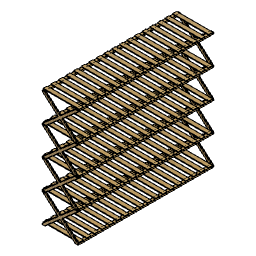
rgiro_akozlin_shelf (Autodesk Fusion 360 design; units mm, degrees)
Autodesk Fusion 360 part; units mm, degrees
note: some values were not read from the file. Chosen so that the rebuilt part matches the saved one: which bodies a step acts on. Set by a fixed rule: which face or edge a step refers to.
sketch "Sketch1" plane through (0, 0, 0) normal (0, 0, 1) x (1, 0, 0)
  line L0 (115, -500) -> (135, -500)
  line L1 (135, -500) -> (135, 500)
  line L2 (135, 500) -> (115, 500)
  line L3 (115, 500) -> (115, -500)
  line L4 (-135, -500) -> (-115, -500)
  line L5 (-115, -500) -> (-115, 500)
  line L6 (-115, 500) -> (-135, 500)
  line L7 (-135, 500) -> (-135, -500)
  dimension "d1" = 270
  dimension "d2" = 1000
  dimension "d4" = 20
  dimension "d7" = 135
  dimension "d29" = 500
  constraint horizontal L0
  constraint vertical L1
  constraint horizontal L2
  constraint vertical L3
  constraint horizontal L4
  constraint vertical L5
  constraint horizontal L6
  constraint vertical L7
  constraint equal L1 L7
  constraint equal L2 L6
  constraint collinear L2 L6
  measures "d1" distance of L1 L7
  measures "d2" distance of L4.start L6.end
  measures "d4" distance of L5.end L6.end
  measures "d7" distance of origin L1
  measures "d29" distance of origin L6
extrude "Extrude1" add sketch "Sketch1" along normal blind 10 makes body 1 at (121.6667, 166.6667, 0) makes body 2 at (-121.6667, 166.6667, 0)
sketch "Sketch2" plane through (0, 0, 10) normal (0, 0, 1) x (-1, 0, 0)
  line L0 (-115, -500) -> (-115, 500)
  line L1 (-115, 500) -> (-135, 500)
  line L2 (-135, 500) -> (-135, -500)
  line L3 (-135, -500) -> (-115, -500)
  line L4 (-135, 500) -> (135, 500)
  line L5 (135, 500) -> (135, 470)
  line L6 (135, 470) -> (-135, 470)
  line L7 (-135, 470) -> (-135, 500)
  line L8 (135, -500) -> (135, 500)
  dimension "d14" = 30
  constraint horizontal L4
  constraint vertical L5
  constraint horizontal L6
  constraint vertical L7
  constraint coincident L1.end L2.start
  constraint collinear L5 L8
  measures "d14" distance of L4.end L5.end
extrude "Extrude2" add sketch "Sketch2" along normal blind 5 separate body contours L0 L1 L2 L4 L6 L7 | L0 L4 L5 L6 L8 makes body 3
pattern_linear "R-Pattern3" count 18 spacing 57.0588 along (0, 1, 0) of bodies 3 makes body 4 at (31.6667, -432.9412, 10) makes body 5 at (31.6667, -375.8824, 10) makes body 6 at (31.6667, -318.8235, 10) makes body 7 at (31.6667, -261.7647, 10) makes body 8 at (31.6667, -204.7059, 10) makes body 9 at (31.6667, -147.6471, 10) makes body 10 at (31.6667, -90.5882, 10) makes body 11 at (31.6667, -33.5294, 10) makes body 12 at (31.6667, 23.5294, 10) makes body 13 at (31.6667, 80.5882, 10) makes body 14 at (31.6667, 137.6471, 10) makes body 15 at (31.6667, 194.7059, 10) makes body 16 at (31.6667, 251.7647, 10) makes body 17 at (31.6667, 308.8235, 10) makes body 18 at (31.6667, 365.8824, 10) makes body 19 at (31.6667, 422.9412, 10) makes body 20 at (31.6667, 480, 10)
pattern_linear "R-Pattern4" count 5 spacing 216.25 along (0, 0, 1) of bodies 8 2 18 16 17 4 14 20 13 1 19 3 11 5 6 12 15 9 10 7 makes body 21 at (31.6667, 365.8824, 226.25) makes body 22 at (31.6667, 365.8824, 442.5) makes body 23 at (31.6667, 365.8824, 658.75) makes body 24 at (31.6667, 365.8824, 875) makes body 25 at (31.6667, -490, 226.25) makes body 26 at (31.6667, -490, 442.5) makes body 27 at (31.6667, -490, 658.75) makes body 28 at (31.6667, -490, 875) makes body 29 at (-121.6667, 166.6667, 216.25) makes body 30 at (-121.6667, 166.6667, 432.5) makes body 31 at (-121.6667, 166.6667, 648.75) makes body 32 at (-121.6667, 166.6667, 865) makes body 33 at (31.6667, 308.8235, 226.25) makes body 34 at (31.6667, 308.8235, 442.5) makes body 35 at (31.6667, 308.8235, 658.75) makes body 36 at (31.6667, 308.8235, 875) makes body 37 at (31.6667, 480, 226.25) makes body 38 at (31.6667, 480, 442.5) makes body 39 at (31.6667, 480, 658.75) makes body 40 at (31.6667, 480, 875) makes body 41 at (31.6667, 23.5294, 226.25) makes body 42 at (31.6667, 23.5294, 442.5) makes body 43 at (31.6667, 23.5294, 658.75) makes body 44 at (31.6667, 23.5294, 875) makes body 45 at (31.6667, 422.9412, 226.25) makes body 46 at (31.6667, 422.9412, 442.5) makes body 47 at (31.6667, 422.9412, 658.75) makes body 48 at (31.6667, 422.9412, 875) makes body 49 at (31.6667, 80.5882, 226.25) makes body 50 at (31.6667, 80.5882, 442.5) makes body 51 at (31.6667, 80.5882, 658.75) makes body 52 at (31.6667, 80.5882, 875) makes body 53 at (31.6667, 137.6471, 226.25) makes body 54 at (31.6667, 137.6471, 442.5) makes body 55 at (31.6667, 137.6471, 658.75) makes body 56 at (31.6667, 137.6471, 875) makes body 57 at (31.6667, 194.7059, 226.25) makes body 58 at (31.6667, 194.7059, 442.5) makes body 59 at (31.6667, 194.7059, 658.75) makes body 60 at (31.6667, 194.7059, 875) makes body 61 at (31.6667, 251.7647, 226.25) makes body 62 at (31.6667, 251.7647, 442.5) makes body 63 at (31.6667, 251.7647, 658.75) makes body 64 at (31.6667, 251.7647, 875) makes body 65 at (121.6667, 166.6667, 216.25) makes body 66 at (121.6667, 166.6667, 432.5) makes body 67 at (121.6667, 166.6667, 648.75) makes body 68 at (121.6667, 166.6667, 865) makes body 69 at (31.6667, -33.5294, 226.25) makes body 70 at (31.6667, -33.5294, 442.5) makes body 71 at (31.6667, -33.5294, 658.75) makes body 72 at (31.6667, -33.5294, 875) makes body 73 at (31.6667, -375.8824, 226.25) makes body 74 at (31.6667, -375.8824, 442.5) makes body 75 at (31.6667, -375.8824, 658.75) makes body 76 at (31.6667, -375.8824, 875) makes body 77 at (31.6667, -318.8235, 226.25) makes body 78 at (31.6667, -318.8235, 442.5) makes body 79 at (31.6667, -318.8235, 658.75) makes body 80 at (31.6667, -318.8235, 875) makes body 81 at (31.6667, -432.9412, 226.25) makes body 82 at (31.6667, -432.9412, 442.5) makes body 83 at (31.6667, -432.9412, 658.75) makes body 84 at (31.6667, -432.9412, 875) makes body 85 at (31.6667, -147.6471, 226.25) makes body 86 at (31.6667, -147.6471, 442.5) makes body 87 at (31.6667, -147.6471, 658.75) makes body 88 at (31.6667, -147.6471, 875) makes body 89 at (31.6667, -90.5882, 226.25) makes body 90 at (31.6667, -90.5882, 442.5) makes body 91 at (31.6667, -90.5882, 658.75) makes body 92 at (31.6667, -90.5882, 875) makes body 93 at (31.6667, -261.7647, 226.25) makes body 94 at (31.6667, -261.7647, 442.5) makes body 95 at (31.6667, -261.7647, 658.75) makes body 96 at (31.6667, -261.7647, 875) makes body 97 at (31.6667, -204.7059, 226.25) makes body 98 at (31.6667, -204.7059, 442.5) makes body 99 at (31.6667, -204.7059, 658.75) makes body 100 at (31.6667, -204.7059, 875)
sketch "Sketch3" plane through (0, 500, 0) normal (0, 1, 0) x (-1, 0, 0)
  line L0 (-135, 0) -> (-115, 0)
  line L1 (-115, 0) -> (-115, 10)
  line L2 (-115, 10) -> (-135, 10)
  line L3 (-135, 10) -> (-135, 0)
  line L4 (-135, 216.25) -> (-115, 216.25)
  line L5 (-115, 216.25) -> (-115, 226.25)
  line L6 (-115, 226.25) -> (-135, 226.25)
  line L7 (-135, 226.25) -> (-135, 216.25)
  line L8 (-135, 226.25) -> (135, 226.25)
  line L9 (135, 226.25) -> (135, 231.25)
  line L10 (135, 231.25) -> (-135, 231.25)
  line L11 (-135, 231.25) -> (-135, 226.25)
  line L12 (115, 216.25) -> (135, 216.25)
  line L13 (135, 216.25) -> (135, 226.25)
  line L14 (135, 226.25) -> (115, 226.25)
  line L15 (115, 226.25) -> (115, 216.25)
  line L16 (115, 10) -> (135, 10)
  line L17 (115, 0) -> (135, 0)
  line L18 (135, 0) -> (135, 10)
  line L19 (135, 10) -> (115, 10)
  line L20 (115, 10) -> (115, 0)
  line L21 (-135, 10) -> (135, 10)
  line L22 (135, 10) -> (135, 15)
  line L23 (135, 15) -> (-135, 15)
  line L24 (-135, 15) -> (-135, 10)
  line L25 (-135, 216.25) -> (115, 0)
  line L26 (-115, 226.25) -> (135, 10)
  line L27 (115, 226.25) -> (-135, 10)
  line L28 (135, 216.25) -> (-115, 0)
  constraint coincident L4.start L7.end
  constraint coincident L17.start L20.end
  constraint coincident L5.end L6.start
  constraint coincident L16.end L18.end
  constraint coincident L14.end L15.start
  constraint coincident L2.end L3.start
  constraint coincident L12.end L13.start
  constraint coincident L0.end L1.start
extrude "Extrude3" add sketch "Sketch3" along normal blind 10 separate body contours L0 L1 L2 L3 L21 | L1 L21 L28 | L2 L21 L23 L27 L28 | L23 L25 L27 L28 | L16 L19 L21 L23 L25 L26 | L20 L21 L25 | L25 L26 L27 L28 | L4 L5 L25 L26 L27 | L16 L17 L18 L19 L20 L21 | L23 L25 L26 L28 | L4 L5 L6 L7 L8 | L12 L15 L26 L27 L28 | L8 L12 L13 L14 L15 makes body 101
fillet "Fillet1" radius 2 18 faces at (80.8863, 500, 47.7083) (80.8863, 510, 47.7083) (-131.1464, 503.3333, 13.3333) (-95.2601, 503.3333, 181.875) (76.6667, 503.3333, 193.0917) (107.2929, 503.3333, 6.6667) (53.5934, 503.3333, 80.4167) (95.2601, 506.6667, 181.875) (-76.6667, 503.3333, 193.0917) (-32.553, 503.3333, 71.3167) (-121.6667, 503.3333, 226.25) (-135, 503.3333, 219.5833) (121.6667, 503.3333, 226.25) (135, 503.3333, 222.9167) (135, 503.3333, 6.6667) (128.3333, 503.3333, 0) (-121.6667, 506.6667, 0) (-135, 503.3333, 3.3333) on bodies 101
pattern_linear "R-Pattern5" count 2 spacing 1010 along (0, -1, 0) count 4 spacing 216.3333 along (0, 0, 1) of bodies 101 makes body 102 at (88.3219, -500, 185.8549) makes body 103 at (-88.3219, 510, 402.1882) makes body 104 at (-88.3219, -500, 402.1882) makes body 105 at (88.3219, 500, 618.5216) makes body 106 at (88.3219, -510, 618.5216) makes body 107 at (-88.3219, 500, 834.8549) makes body 108 at (-88.3219, -510, 834.8549)
